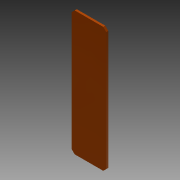
# Autodesk Inventor part: multiplier_pcb
Saved by Autodesk Inventor 2015 (Build 190159000, 159)
## iProperties
Created: 2014-10-08
Part Number: multiplier_pcb
Material: Phenolic Resin
Document SubType Name: Modeling
Designer: Adam
Density: 1.38 g/cm^3
Appearance: Smooth - Light Orange
Author: Adam
Autodesk Inventor part; units mm, degrees
ref_plane "YZ Plane" through (0, 0, 0) normal (1, 0, 0) x (0, 1, 0)
ref_plane "XZ Plane" through (0, 0, 0) normal (0, 1, 0) x (-1, 0, 0)
ref_plane "XY Plane" through (0, 0, 0) normal (0, 0, 1) x (1, 0, 0)
sketch "Sketch1" plane through (0, 0, 0) normal (0, 0, 1) x (1, 0, 0)
  arc A0 (6.9595, 53) -> (8.4595, 54.5) centre (6.9595, 54.5) ccw projected
  line L0 (1.4595, 54.5) -> (8.4595, 54.5) projected
  arc A1 (1.4595, 54.5) -> (-1.5405, 51.5) centre (1.4595, 51.5) ccw projected
  line L1 (-1.5405, -51.5) -> (-1.5405, 51.5) projected
  arc A2 (-1.5405, -51.5) -> (1.4595, -54.5) centre (1.4595, -51.5) ccw projected
  line L2 (8.4595, -54.5) -> (1.4595, -54.5) projected
  arc A3 (8.4595, -54.5) -> (6.9595, -53) centre (6.9595, -54.5) ccw projected
  line L3 (1.4595, -53) -> (6.9595, -53) projected
  arc A4 (-0.0405, -51.5) -> (1.4595, -53) centre (1.4595, -51.5) ccw projected
  line L4 (-0.0405, 51.5) -> (-0.0405, -51.5) projected
  arc A5 (1.4595, 53) -> (-0.0405, 51.5) centre (1.4595, 51.5) ccw projected
  line L5 (6.9595, 53) -> (1.4595, 53) projected
  arc A6 (1.4595, 54.1) -> (-1.1405, 51.5) centre (1.4595, 51.5) ccw construction
  line L6 (1.4595, 54.1) -> (26.2595, 54.1)
  line L7 (-1.1405, 51.5) -> (-1.1405, -51.5)
  arc A7 (-1.1405, -51.5) -> (1.4595, -54.1) centre (1.4595, -51.5) ccw construction
  line L8 (1.4595, -54.1) -> (26.2595, -54.1)
  line L9 (-1.1405, -51.5) -> (1.4595, -54.1)
  line L10 (1.4595, 54.1) -> (-1.1405, 51.5)
  line L11 (26.2595, 54.1) -> (28.8595, 51.5)
  line L12 (28.8595, 51.5) -> (28.8595, -51.5)
  line L13 (28.8595, -51.5) -> (26.2595, -54.1)
  point P0 (0, 0)
  dimension "d0" = 0.4
  dimension "d1" = 30
  constraints: 16 end point, 5 point on circle, 4 tangent, 2 centre point, 2 coincident, 2 horizontal, 2 horizontal alignment, 2 perpendicular, 2 vertical, 1 vertical alignment
  measures "d0" radial gap between concentric circles of A1 A6
  measures "d1" distance between parallel lines of L7 L12
extrude "Extrusion1" add sketch "Sketch1" along normal blind 1.8 contours L5 A5 L4 A4 L3 A3 L8 L9 L7 L10 L6 A0 | A0 L6 L11 L12 L13 L8 A3 L3 A4 L4 A5 L5
body "Solid1"
